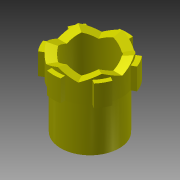
# Autodesk Inventor part: Pulsador
Saved by Autodesk Inventor 2014 (Build 180170000, 170)
## iProperties
Created: 2017-02-07
Part Number: Pulsador
Material: Generic
Document SubType Name: Modeling
Designer: Rubén
Density: 1 g/cm^3
Appearance: Smooth - Yellow
Author: Rubén
Autodesk Inventor part; units mm, degrees
ref_plane "YZ Plane" through (0, 0, 0) normal (1, 0, 0) x (0, 1, 0)
ref_plane "XZ Plane" through (0, 0, 0) normal (0, 1, 0) x (-1, 0, 0)
ref_plane "XY Plane" through (0, 0, 0) normal (0, 0, 1) x (1, 0, 0)
sketch "Sketch1" plane through (0, 0, 0) normal (0, 1, 0) x (-1, 0, 0)
  circle A0 centre (0, 0) radius 4.75
  dimension "d0" = 9.5
  constraints: 1 centre point, 1 coincident
  measures "d0" diameter of A0
sketch "Sketch1 outline for Extrusion1" plane through (0, 0, 0) normal (0, 1, 0) x (-1, 0, 0)
  circle A0 centre (0, 0) radius 4.75
extrude "Extrusion1" add sketch "Sketch1 outline for Extrusion1" along normal blind 10
sketch "Sketch2" plane through (0, 10, 0) normal (0, 1, 0) x (1, 0, 0)
  circle A0 centre (0, 0) radius 4.75
  circle A1 centre (0, 0) radius 5.25
  arc A2 (1.1, 5.898305) -> (-1.1, 5.898305) centre (0, 0) ccw
  line L0 (0, 6) -> (0, 0) construction
  line L1 (-1.1, 5.898305) -> (-1.1, 5.133469)
  line L2 (1.1, 5.898305) -> (1.1, 5.133469)
  arc A3 (1.1, 5.133469) -> (-1.1, 5.133469) centre (0, 0) ccw
  arc A4 (-4.558082, 3.90178) -> (-5.658082, 1.996524) centre (0, 0) ccw
  line L3 (-5.658082, 1.996524) -> (-4.995714, 1.614106)
  line L4 (-4.558082, 3.90178) -> (-3.895714, 3.519362)
  arc A5 (-3.895714, 3.519362) -> (-4.995714, 1.614106) centre (0, 0) ccw
  arc A6 (-5.658082, -1.996524) -> (-4.558082, -3.90178) centre (0, 0) ccw
  line L5 (-4.558082, -3.90178) -> (-3.895714, -3.519362)
  line L6 (-5.658082, -1.996524) -> (-4.995714, -1.614106)
  arc A7 (-4.995714, -1.614106) -> (-3.895714, -3.519362) centre (0, 0) ccw
  arc A8 (-1.1, -5.898305) -> (1.1, -5.898305) centre (0, 0) ccw
  line L7 (1.1, -5.898305) -> (1.1, -5.133469)
  line L8 (-1.1, -5.898305) -> (-1.1, -5.133469)
  arc A9 (-1.1, -5.133469) -> (1.1, -5.133469) centre (0, 0) ccw
  arc A10 (4.558082, -3.90178) -> (5.658082, -1.996524) centre (0, 0) ccw
  line L9 (5.658082, -1.996524) -> (4.995714, -1.614106)
  line L10 (4.558082, -3.90178) -> (3.895714, -3.519362)
  arc A11 (3.895714, -3.519362) -> (4.995714, -1.614106) centre (0, 0) ccw
  arc A12 (5.658082, 1.996524) -> (4.558082, 3.90178) centre (0, 0) ccw
  line L11 (4.558082, 3.90178) -> (3.895714, 3.519362)
  line L12 (5.658082, 1.996524) -> (4.995714, 1.614106)
  arc A13 (4.995714, 1.614106) -> (3.895714, 3.519362) centre (0, 0) ccw
  point P0 (-5.196152, 3)
  point P1 (-5.196152, -3)
  point P2 (0, -6)
  point P3 (5.196152, -3)
  point P4 (5.196152, 3)
  dimension "d3" = 10.5
  dimension "d6" = 2.2
  dimension "d7" = 6
  dimension "d10" = 360
  constraints: 27 point on circle, 26 end point, 13 centre point, 10 coincident, 2 parallel, 1 vertical, 65 other
  measures "d3" diameter of A1
  measures "d6" distance between parallel lines of L2 L1
  measures "d7" radius of A2
sketch "Sketch2 outline for Extrusion2" plane through (0, 10, 0) normal (0, 1, 0) x (1, 0, 0)
  line L0 (1.1, 5.133469) -> (1.1, 5.898305)
  arc A0 (1.1, 5.898305) -> (-1.1, 5.898305) centre (0, 0) ccw
  line L1 (-1.1, 5.898305) -> (-1.1, 5.133469)
  arc A1 (-1.1, 5.133469) -> (-3.895714, 3.519362) centre (0, 0) ccw
  line L2 (-3.895714, 3.519362) -> (-4.558082, 3.90178)
  arc A2 (-4.558082, 3.90178) -> (-5.658082, 1.996524) centre (0, 0) ccw
  line L3 (-5.658082, 1.996524) -> (-4.995714, 1.614106)
  arc A3 (-4.995714, 1.614106) -> (-4.995714, -1.614106) centre (0, 0) ccw
  line L4 (-4.995714, -1.614106) -> (-5.658082, -1.996524)
  arc A4 (-5.658082, -1.996524) -> (-4.558082, -3.90178) centre (0, 0) ccw
  line L5 (-4.558082, -3.90178) -> (-3.895714, -3.519362)
  arc A5 (-3.895714, -3.519362) -> (-1.1, -5.133469) centre (0, 0) ccw
  line L6 (-1.1, -5.133469) -> (-1.1, -5.898305)
  arc A6 (-1.1, -5.898305) -> (1.1, -5.898305) centre (0, 0) ccw
  line L7 (1.1, -5.898305) -> (1.1, -5.133469)
  arc A7 (1.1, -5.133469) -> (3.895714, -3.519362) centre (0, 0) ccw
  line L8 (3.895714, -3.519362) -> (4.558082, -3.90178)
  arc A8 (4.558082, -3.90178) -> (5.658082, -1.996524) centre (0, 0) ccw
  line L9 (5.658082, -1.996524) -> (4.995714, -1.614106)
  arc A9 (4.995714, -1.614106) -> (4.995714, 1.614106) centre (0, 0) ccw
  line L10 (4.995714, 1.614106) -> (5.658082, 1.996524)
  arc A10 (5.658082, 1.996524) -> (4.558082, 3.90178) centre (0, 0) ccw
  line L11 (4.558082, 3.90178) -> (3.895714, 3.519362)
  arc A11 (3.895714, 3.519362) -> (1.1, 5.133469) centre (0, 0) ccw
  circle A12 centre (0, 0) radius 4.75
extrude "Extrusion2" add sketch "Sketch2 outline for Extrusion2" against normal blind 2.5
sketch "Sketch3" plane through (0, 10, 0) normal (0, 1, 0) x (1, 0, 0)
  arc A0 (1.1, -5.133469) -> (3.895714, -3.519362) centre (0, 0) ccw
  circle A1 centre (0, 0) radius 3.8
  dimension "d12" = 7.6
  constraints: 1 centre point, 1 coincident
  measures "d12" diameter of A1
sketch "Sketch3 outline for Extrusion3" plane through (0, 10, 0) normal (0, 1, 0) x (1, 0, 0)
  circle A0 centre (0, 0) radius 3.8
extrude "Extrusion3" cut sketch "Sketch3 outline for Extrusion3" against normal blind 8.5
sketch "Sketch5" plane through (0, 10, 0) normal (0, 1, 0) x (1, 0, 0)
  circle A0 centre (0, 0) radius 3.8
  arc A1 (1.1, 5.898305) -> (-1.1, 5.898305) centre (0, 0) ccw
  line L0 (-1.1, 5.898305) -> (-1.1, 5.133469)
  arc A2 (-1.1, 5.133469) -> (-3.895714, 3.519362) centre (0, 0) ccw
  line L1 (1.1, -5.898305) -> (1.1, -5.133469)
  arc A3 (1.1, -5.133469) -> (3.895714, -3.519362) centre (0, 0) ccw
  line L2 (0, 6) -> (0, 5.25) construction
  line L3 (0, 0) -> (-1.9, 3.290897) construction
  line L4 (-1.9, 3.290897) -> (-2.625, 4.546633)
  arc A4 (-1.1, -5.898305) -> (1.1, -5.898305) centre (0, 0) ccw
  arc A5 (0, 5.25) -> (-1.1, 5.133469) centre (0, 0) ccw
  line L5 (0, 5.25) -> (0, 3.8)
  constraints: 8 end point, 6 point on circle, 2 parallel, 1 centre point, 1 coincident, 1 line through centre
sketch "Sketch5 outline for Extrusion4" plane through (0, 10, 0) normal (0, 1, 0) x (1, 0, 0)
  arc A0 (0, 5.25) -> (-1.1, 5.133469) centre (0, 0) ccw
  line L0 (0, 3.8) -> (0, 5.25)
  arc A1 (-1.9, 3.290897) -> (0, 3.8) centre (0, 0) cw
  line L1 (-2.625, 4.546633) -> (-1.9, 3.290897)
  arc A2 (-1.1, 5.133469) -> (-2.625, 4.546633) centre (0, 0) ccw
extrude "Extrusion4" add sketch "Sketch5 outline for Extrusion4" along normal blind 0.5
draft "FaceDraft1" angle 25 pull direction (-0.8660254, 0, 0.5) faces at (-1.779226, 10.5, -3.885556) fixed edges at (-2.2625, 10.5, -3.918765)
mirror "Mirror1" about plane through (0, 10, -3.8) normal (1, 0, 0) of "Extrusion4", "FaceDraft1"
pattern_circular "Circular Pattern1" count 6 over 360 about axis through (0, 10, 0) along (0, -1, 0) of "Extrusion4", "FaceDraft1", "Mirror1"
sketch "Sketch6" plane through (0, 10, 0) normal (0, 1, 0) x (1, 0, 0)
  arc A0 (1.1, 5.133469) -> (-1.1, 5.133469) centre (0, 0) ccw
  line L0 (1.1, 5.133469) -> (1.1, 5.898305)
  arc A1 (1.1, 5.898305) -> (-1.1, 5.898305) centre (0, 0) ccw
  line L1 (-1.1, 5.898305) -> (-1.1, 5.133469)
  arc A2 (4.995714, 1.614106) -> (3.895714, 3.519362) centre (0, 0) ccw
  line L2 (4.995714, 1.614106) -> (5.658082, 1.996524)
  arc A3 (5.658082, 1.996524) -> (4.558082, 3.90178) centre (0, 0) ccw
  line L3 (4.558082, 3.90178) -> (3.895714, 3.519362)
  arc A4 (3.895714, -3.519362) -> (4.995714, -1.614106) centre (0, 0) ccw
  line L4 (3.895714, -3.519362) -> (4.558082, -3.90178)
  arc A5 (4.558082, -3.90178) -> (5.658082, -1.996524) centre (0, 0) ccw
  line L5 (5.658082, -1.996524) -> (4.995714, -1.614106)
  arc A6 (-1.1, -5.133469) -> (1.1, -5.133469) centre (0, 0) ccw
  line L6 (-1.1, -5.133469) -> (-1.1, -5.898305)
  arc A7 (-1.1, -5.898305) -> (1.1, -5.898305) centre (0, 0) ccw
  line L7 (1.1, -5.898305) -> (1.1, -5.133469)
  arc A8 (-4.995714, -1.614106) -> (-3.895714, -3.519362) centre (0, 0) ccw
  line L8 (-4.995714, -1.614106) -> (-5.658082, -1.996524)
  arc A9 (-5.658082, -1.996524) -> (-4.558082, -3.90178) centre (0, 0) ccw
  line L9 (-4.558082, -3.90178) -> (-3.895714, -3.519362)
  arc A10 (-3.895714, 3.519362) -> (-4.995714, 1.614106) centre (0, 0) ccw
  line L10 (-3.895714, 3.519362) -> (-4.558082, 3.90178)
  arc A11 (-4.558082, 3.90178) -> (-5.658082, 1.996524) centre (0, 0) ccw
  line L11 (-5.658082, 1.996524) -> (-4.995714, 1.614106)
sketch "Sketch6 outline for Extrusion5" plane through (0, 10, 0) normal (0, 1, 0) x (1, 0, 0)
  line L0 (-1.1, 5.898305) -> (-1.1, 5.133469)
  arc A0 (1.1, 5.898305) -> (-1.1, 5.898305) centre (0, 0) ccw
  line L1 (1.1, 5.133469) -> (1.1, 5.898305)
  arc A1 (-1.1, 5.133469) -> (1.1, 5.133469) centre (0, 0) cw
  line L2 (4.558082, 3.90178) -> (3.895714, 3.519362)
  arc A2 (5.658082, 1.996524) -> (4.558082, 3.90178) centre (0, 0) ccw
  line L3 (4.995714, 1.614106) -> (5.658082, 1.996524)
  arc A3 (3.895714, 3.519362) -> (4.995714, 1.614106) centre (0, 0) cw
  line L4 (5.658082, -1.996524) -> (4.995714, -1.614106)
  arc A4 (4.558082, -3.90178) -> (5.658082, -1.996524) centre (0, 0) ccw
  line L5 (3.895714, -3.519362) -> (4.558082, -3.90178)
  arc A5 (4.995714, -1.614106) -> (3.895714, -3.519362) centre (0, 0) cw
  line L6 (1.1, -5.898305) -> (1.1, -5.133469)
  arc A6 (-1.1, -5.898305) -> (1.1, -5.898305) centre (0, 0) ccw
  line L7 (-1.1, -5.133469) -> (-1.1, -5.898305)
  arc A7 (1.1, -5.133469) -> (-1.1, -5.133469) centre (0, 0) cw
  line L8 (-4.558082, -3.90178) -> (-3.895714, -3.519362)
  arc A8 (-5.658082, -1.996524) -> (-4.558082, -3.90178) centre (0, 0) ccw
  line L9 (-4.995714, -1.614106) -> (-5.658082, -1.996524)
  arc A9 (-3.895714, -3.519362) -> (-4.995714, -1.614106) centre (0, 0) cw
  line L10 (-5.658082, 1.996524) -> (-4.995714, 1.614106)
  arc A10 (-4.558082, 3.90178) -> (-5.658082, 1.996524) centre (0, 0) ccw
  line L11 (-3.895714, 3.519362) -> (-4.558082, 3.90178)
  arc A11 (-4.995714, 1.614106) -> (-3.895714, 3.519362) centre (0, 0) cw
extrude "Extrusion5" add sketch "Sketch6 outline for Extrusion5" along normal blind 1
body "Solid1"
